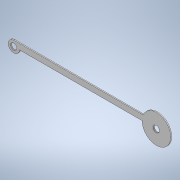
# Autodesk Inventor part: Pieza6
Saved by Autodesk Inventor 2022 (Build 260153000, 153)
## iProperties
Created: 2022-11-04
Part Number: Pieza6
Material: Genérico
Document SubType Name: Modeling
Designer: Mauricio Guerrero
Density: 1 g/cm^3
Appearance: Valor por defecto
Author: Mauricio Guerrero
Autodesk Inventor part; units mm, degrees
ref_plane "YZ Plane" through (0, 0, 0) normal (1, 0, 0) x (0, 1, 0)
ref_plane "XZ Plane" through (0, 0, 0) normal (0, 1, 0) x (-1, 0, 0)
ref_plane "XY Plane" through (0, 0, 0) normal (0, 0, 1) x (1, 0, 0)
sketch "Boceto1" plane through (0, 0, 0) normal (0, 0, 1) x (1, 0, 0)
  circle A0 centre (-1129.4428, 209.4977) radius 1.25
  arc A1 (-1129.4428, 211.7327) -> (-1127.2078, 209.5027) centre (-1129.4428, 209.4977) ccw
  circle A2 centre (-1072.2928, 209.4977) radius 1.25
  arc A3 (-1078.0328, 209.5027) -> (-1077.5798, 211.7327) centre (-1072.2928, 209.4977) ccw
  line L0 (-1129.4428, 211.7327) -> (-1077.5798, 211.7327)
  line L1 (-1129.1407, 209.5027) -> (-1128.1928, 209.5027)
  line L2 (-1127.2078, 209.5027) -> (-1078.0328, 209.5027)
  dimension "d9" = 4.47
  dimension "d10" = 2.5
  dimension "d12" = 11.48
  dimension "d16" = 57.15
  constraints: 6 end point, 4 point on circle, 3 centre point, 3 horizontal, 2 coincident, 1 horizontal alignment, 1 tangent, 3 other
  measures "d9" diameter of A1
  measures "d10" diameter of A2
  measures "d12" diameter of A3
  measures "d16" distance of A2.centre point (-1129.443, 209.498)
extrude "Extrusión1" add sketch "Boceto1" along normal blind 0.4
